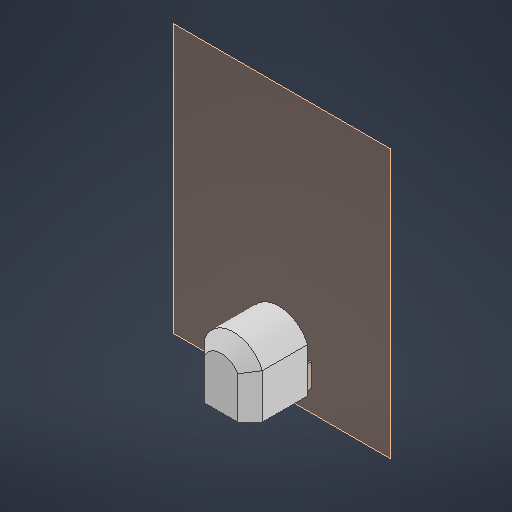
# Autodesk Inventor part: lid
Saved by Autodesk Inventor 2026.1 (Build 301233000, 233)
## iProperties
Created: 2025-08-20
Part Number: lid
Material: Generic
Document SubType Name: Modeling
Designer: mateo
Density: 1 g/cm^3
Appearance: Default
Author: mateo
Autodesk Inventor part; units mm, degrees
ref_plane "YZ Plane" through (0, 0, 0) normal (1, 0, 0) x (0, 1, 0)
ref_plane "XZ Plane" through (0, 0, 0) normal (0, 1, 0) x (-1, 0, 0)
ref_plane "XY Plane" through (0, 0, 0) normal (0, 0, 1) x (1, 0, 0)
ref_plane "Work Plane1" through (0, 0, -19.1344) normal (0, 0, 1) x (1, 0, 0)
sketch "Sketch1" plane through (0, 0, -19.1344) normal (0, 0, 1) x (1, 0, 0)
  line L0 (25.2444, -123.4114) -> (25.2444, -170.4025) projected
  line L1 (-32.7556, -123.4114) -> (-32.7556, -170.4025) projected
  line L2 (-32.7556, -170.4025) -> (25.2444, -170.4025) projected
  arc A0 (25.2444, -123.4114) -> (-32.7556, -123.4114) centre (-3.7556, -136.9392) ccw projected
  line L3 (31.2444, -121.7507) -> (31.2444, -177.7298) projected
  line L4 (31.2444, -177.7298) -> (25.2444, -184.0804) projected
  line L5 (25.2444, -184.0804) -> (-32.7556, -184.0804) projected
  line L6 (-38.7556, -121.7507) -> (-38.7556, -177.7298) projected
  arc A1 (31.2444, -137.3523) -> (-38.7556, -137.3523) centre (-3.7556, -6.9683) ccw projected
  line L7 (-38.7556, -176.4025) -> (-38.7556, -122.1405)
  arc A2 (31.2444, -122.1405) -> (-38.7556, -122.1405) centre (-3.7556, -136.9392) ccw
  line L8 (31.2444, -122.1405) -> (31.2444, -176.4025)
  line L9 (31.2444, -176.4025) -> (-38.7556, -176.4025)
  line L10 (-34.1735, -168.01) -> (-34.1735, -172.796)
  line L11 (-34.1735, -172.796) -> (-28.1735, -179.1467)
  point P0 (0, 0)
  point P1 (31.2444, -122.1405)
  point P2 (-38.7556, -122.1405)
  point P3 (31.2444, -176.4025)
  point P4 (31.2444, -122.1405)
  point P5 (-28.1735, -165.4687)
  point P6 (-34.1735, -171.4687)
  point P7 (-38.7556, -176.4025)
  point P8 (-34.1735, -171.4687)
  point P9 (-28.1735, -179.1467)
  dimension "d1" = 0
  constraints: 10 end point, 2 point on circle, 1 centre point, 3 other
  measures "d1" distance between parallel lines of L6 L7
extrude "Extrusion1" add sketch "Sketch1" along normal blind 70 contours L0 L2 L1 A0 | L3 L9 L6 A2
shell "Shell2" thickness 6 removed faces 2 at (7.9111, -158.3152, -19.1344) at (-15.4223, -176.4025, 4.1989)
sketch "Sketch4" plane through (0, 0, -19.1344) normal (0, 0, -1) x (-1, 0, 0)
  line L0 (37.0056, -172.4025) -> (34.5056, -172.4025)
  line L1 (34.5056, -172.4025) -> (34.5056, -162.4025)
  line L2 (37.0056, -162.4025) -> (37.0056, -172.4025)
  line L3 (34.5056, -154.4025) -> (34.5056, -144.4025)
  line L4 (34.5056, -144.4025) -> (37.0056, -144.4025)
  line L5 (37.0056, -144.4025) -> (37.0056, -154.4025)
  line L6 (38.7556, -176.4025) -> (32.7556, -176.4025) projected
  line L7 (32.7556, -176.4025) -> (-25.2444, -176.4025) projected
  line L8 (3.7556, -176.4025) -> (3.7556, -125.4125)
  line L9 (-29.4944, -172.4025) -> (-26.9944, -172.4025)
  line L10 (-26.9944, -172.4025) -> (-26.9944, -162.4025)
  line L11 (-29.4944, -162.4025) -> (-29.4944, -172.4025)
  line L12 (-26.9944, -154.4025) -> (-26.9944, -144.4025)
  line L13 (-26.9944, -144.4025) -> (-29.4944, -144.4025)
  line L14 (-29.4944, -144.4025) -> (-29.4944, -154.4025)
  line L15 (-31.2444, -176.4025) -> (-25.2444, -176.4025)
  line L16 (37.0056, -154.4025) -> (37.0056, -162.4025)
  line L17 (34.5056, -162.4025) -> (34.5056, -154.4025)
  line L18 (-26.9944, -154.4025) -> (-26.9944, -163.1669)
  line L19 (-29.4944, -154.4025) -> (-29.4944, -163.8854)
  line L20 (38.7556, -122.1405) -> (38.7556, -176.4025) projected
  line L21 (32.7556, -123.4114) -> (32.7556, -176.4025) projected
  point P0 (0, 0)
  point P1 (18.2703, -176.4025)
  point P2 (-10.7591, -176.4025)
  dimension "d60" = 10
  dimension "d61" = 10
  dimension "d63" = 4
  dimension "d77" = 1.75
  dimension "d79" = 1.75
  dimension "d80" = 2.5
  constraints: 36 end point, 10 symmetric about line, 6 point on line, 2 collinear, 2 parallel, 1 horizontal, 1 midpoint, 1 perpendicular, 1 vertical
  measures "d60" distance of L0.end L1.end
  measures "d61" distance of L3.start L3.end
  measures "d63" distance between parallel lines of L0 L6
  measures "d77" distance between parallel lines of L20 L2
  measures "d79" distance between parallel lines of L21 L17
  measures "d80" distance of L3.end L4.end
extrude "Extrusion4" add sketch "Sketch4" along normal blind 7
chamfer "Chamfer6" distance 15 angle 45 3 edges at (-3.7556, -104.9392, 44.8656) (25.2444, -149.9069, 44.8656) (-32.7556, -149.9069, 44.8656)
chamfer "Chamfer7" distance 15 angle 45 3 edges at (-38.7556, -149.2715, 50.8656) (-3.7556, -98.9392, 50.8656) (31.2444, -149.2715, 50.8656)
body "Solid1"
